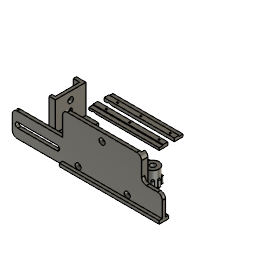
camera_steady (Autodesk Fusion 360 design; units mm, degrees)
Autodesk Fusion 360 part; units mm, degrees
note: some values were not read from the file. Chosen so that the rebuilt part matches the saved one: which face or edge a step refers to; which sketch regions a step uses; which pieces of a blend or face edit are solid.
sketch "Sketch1" plane through (0, 0, 0) normal (0, 0, 1) x (1, 0, 0)
  line L0 (-42, 80) -> (-26, 80)
  line L1 (0, 50) -> (118, 50)
  line L2 (118, 50) -> (118, 62)
  line L3 (118, 62) -> (-70, 62)
  line L4 (-70, 62) -> (-70, 54)
  line L5 (-7, 54) -> (-7, 62)
  line L6 (-3, 54) -> (-3, 62)
  line L7 (88, 50) -> (88, 62)
  line L8 (92, 50) -> (92, 62)
  line L9 (118, 58) -> (-70.000001, 58)
  line L10 (-70, 54) -> (98, 54)
  line L11 (-42, 118.4) -> (-42, 80)
  line L12 (-26, 118.4) -> (-26, 80)
  line L13 (-42, 118.4) -> (-26, 118.4)
  line L14 (-42, 118.4) -> (-46, 118.4)
  line L15 (-42, 80) -> (-46, 80)
  line L16 (-46, 114.4) -> (-46, 84)
  line L17 (-46, 118.4) -> (-54, 118.4)
  line L18 (-46, 80) -> (-50, 80)
  line L19 (-46, 114.4) -> (-54, 114.4)
  line L20 (-46, 80) -> (-50, 80)
  line L21 (-46, 84) -> (-50, 84)
  line L22 (-54, 118.4) -> (-54, 114.4)
  line L23 (-50, 80) -> (-50, 84)
  line L24 (25, 80) -> (50, 80)
  line L25 (50, 80) -> (50, 110)
  line L26 (50, 110) -> (25, 110)
  line L27 (25, 84) -> (50, 84)
  circle A0 centre (35, 95) radius 3.2
  circle A1 centre (35, 95) radius 10.7
  line L28 (-50, 130) -> (36, 130)
  line L29 (36, 141) -> (-50, 141)
  line L30 (-50, 141) -> (-50, 130)
  line L31 (-50, 135) -> (36, 135)
  circle A2 centre (-36.000001, 138.000002) radius 1.1
  circle A3 centre (-7, 138) radius 1.1
  circle A4 centre (30, 138.000002) radius 1.1
  line L32 (-50.000001, 145.000002) -> (35.000001, 145.000002) construction
  circle A5 centre (30, 152.000002) radius 1.1
  line L33 (-50, 149.000004) -> (-50, 160.000004)
  line L34 (-50, 155.000004) -> (36, 155.000004)
  line L35 (36, 149.000004) -> (-50, 149.000004)
  circle A6 centre (-36.000001, 152.000002) radius 1.1
  line L36 (-50, 160.000004) -> (36, 160.000004)
  circle A7 centre (-7, 152.000004) radius 1.1
  line L37 (-44, 141) -> (-44, 130)
  line L38 (-44, 149.000004) -> (-44, 160.000004)
  line L39 (98, 54) -> (118, 54)
  line L40 (20.07966, 95) -> (20.07966, 110)
  line L41 (20.07966, 95) -> (20.07966, 80)
  line L42 (25, 80) -> (20.07966, 80)
  line L43 (25, 84) -> (20.07966, 84)
  line L44 (25, 110) -> (20.07966, 110)
  line L45 (-7, 54) -> (-7, 50)
  line L46 (-7, 50) -> (0, 50)
  circle A8 centre (70.000001, 90.000001) radius 3.3
  circle A9 centre (70.000001, 90.000001) radius 8
  arc A10 (65.498572, 96.613407) -> (63.386595, 94.50143) centre (64.343147, 95.656856) ccw
  arc A11 (71.493395, 97.859376) -> (68.506607, 97.859376) centre (70.000001, 98.000001) ccw
  arc A12 (76.613407, 94.50143) -> (74.50143, 96.613407) centre (75.656855, 95.656856) ccw
  arc A13 (77.859376, 88.506608) -> (77.859376, 91.493395) centre (78.000001, 90.000001) ccw
  arc A14 (74.50143, 83.386595) -> (76.613407, 85.498573) centre (75.656855, 84.343147) ccw
  arc A15 (68.506607, 82.140626) -> (71.493395, 82.140626) centre (70.000001, 82.000001) ccw
  arc A16 (63.386595, 85.498573) -> (65.498572, 83.386595) centre (64.343147, 84.343147) ccw
  arc A17 (62.140626, 91.493395) -> (62.140626, 88.506608) centre (62.000001, 90.000001) ccw
  line L47 (38, 160.000004) -> (38, 149.000004)
  line L48 (36, 149.000004) -> (38, 149.000004)
  line L49 (36, 160.000004) -> (38, 160.000004)
  line L50 (36, 155.000004) -> (38.000001, 155.000004)
  line L51 (38, 130) -> (38, 141)
  line L52 (36, 130) -> (38, 130)
  line L53 (36, 141) -> (38, 141)
  line L54 (36, 135) -> (38, 135)
  line L55 (34.999999, 89.157067) -> (29.939871, 92.078534)
  line L56 (29.939871, 92.078534) -> (29.939872, 97.921467)
  line L57 (29.939872, 97.921467) -> (35.000001, 100.842933)
  line L58 (35.000001, 100.842933) -> (40.060129, 97.921466)
  line L59 (40.060129, 97.921466) -> (40.060128, 92.078533)
  line L60 (40.060128, 92.078533) -> (34.999999, 89.157067)
  point P0 (35, 95)
  point P1 (-7, 141)
  point P2 (-7, 138)
  point P3 (-36.000001, 138.000002)
  point P4 (30, 138.000002)
  point P5 (30, 152.000002)
  point P6 (-7, 152.000004)
  point P7 (-36.000001, 152.000002)
  point P8 (-7, 149.000004)
  point P9 (-44, 130)
  point P10 (-44, 149.000004)
  point P11 (70.000001, 90.000001)
  point P12 (70.000001, 98.000001)
  dimension "d43" = 168
  dimension "d54" = 38.4
  dimension "d64" = 4
  dimension "d69" = 4
  dimension "d81" = 6.4
  dimension "d82" = 21.4
  dimension "d92" = 86
  dimension "d93" = 11
  dimension "d100" = 2.2
  dimension "d101" = 2.2
  dimension "d102" = 2.2
  dimension "d103" = 11
  dimension "d118" = 6.6
  dimension "d119" = 16
  dimension "d120" = 3
  dimension "d122" = 360
  constraint horizontal L0
  constraint horizontal L1
  constraint vertical L2
  constraint horizontal L3
  constraint vertical L4
  constraint coincident L3 L5.end
  constraint perpendicular L3 L5
  constraint coincident L3 L6.end
  constraint perpendicular L3 L6
  constraint coincident L3 L7.end
  constraint perpendicular L3 L7
  constraint coincident L3 L8.end
  constraint perpendicular L3 L8
  constraint coincident L1 L7.start
  constraint coincident L1 L8.start
  constraint horizontal L9
  constraint horizontal L10
  constraint vertical L11
  constraint vertical L12
  constraint coincident L10 L5.start
  constraint perpendicular L12 L13
  constraint perpendicular L11 L14
  constraint perpendicular L11 L15
  constraint perpendicular L16 L17
  constraint perpendicular L16 L18
  constraint perpendicular L19 L22
  constraint perpendicular L21 L23
  constraint horizontal L24
  constraint vertical L25
  constraint horizontal L26
  constraint horizontal L27
  constraint coincident P0 A0.centre
  constraint concentric A0 A1
  constraint horizontal L28
  constraint horizontal L29
  constraint vertical L30
  constraint horizontal L31
  constraint midpoint L29 P1
  constraint coincident P2 A3.centre
  constraint horizontal L32
  constraint symmetric A2 L32 A6
  constraint symmetric A3 L32 A7
  constraint symmetric A4 L32 A5
  constraint vertical L37
  constraint coincident P9 L37.end
  constraint coincident L2 L39.end
  constraint perpendicular L2 L39
  constraint perpendicular L41 L42
  constraint perpendicular L41 L43
  constraint perpendicular L40 L44
  constraint perpendicular L10 L45
  constraint perpendicular L6 L46
  constraint coincident L10 L6.start
  constraint concentric A8 A9
  constraint perpendicular L47 L48
  constraint perpendicular L47 L49
  constraint perpendicular L47 L50
  constraint vertical L51
  constraint perpendicular L51 L52
  constraint perpendicular L51 L53
  constraint coincident L51 L54.end
  constraint perpendicular L51 L54
  measures "d43" distance of L10.end L4.end
  measures "d54" distance of L0.start L11.start
  measures "d64" distance of L0.start L15.end
  measures "d69" distance of L21.end L16.end
  measures "d81" diameter of A0
  measures "d82" diameter of A1
  measures "d92" distance of L28.start L28.end
  measures "d93" distance of L28.start L29.end
  measures "d100" diameter of A2
  measures "d101" diameter of A3
  measures "d102" diameter of A4
  measures "d103" distance of P9 L37.start
  measures "d118" diameter of A8
  measures "d119" diameter of A9
  measures "d120" diameter of A11
extrude "Extrude15" add sketch "Sketch1" along normal blind 4 contours L1 L7 L10 L45 L46 | L1 L7 L8 L10 | L1 L2 L8 L10 L39 | L6 L7 L9 L10 picked at (28.333333, 52.666667) picked at (90.666667, 51.333333) picked at (102.666667, 51.333333) picked at (57.666667, 55.333333) makes body 1
extrude "Extrude16" add sketch "Sketch1" along normal blind 30 contours L4 L5 L9 L10 | L2 L8 L9 L10 L39 picked at (-49, 56.666667) picked at (102.666667, 56.666667) bodies 1
extrude "Extrude31" add sketch "Sketch1" along normal blind 60 contours L6 L7 L9 L10 | L7 L8 L9 L10 | L5 L6 L9 L10 | L3 L7 L8 L9 | L3 L5 L6 L9 picked at (57.666667, 55.333333) picked at (89.333333, 56.666667) picked at (-5.666667, 55.333333) picked at (89.333333, 60.666667) picked at (-5.666667, 59.333333) bodies 1
extrude "Extrude17" add sketch "Sketch1" along normal blind 4 contours L3 L6 L7 L9 | L3 L4 L5 L9 | L2 L3 L8 L9 picked at (57.666667, 59.333333) picked at (-49, 59.333333) picked at (100.666667, 59.333333) bodies 1
sketch "Sketch2" plane through (0, 54, 0) normal (0, -1, 0) x (1, 0, 0)
  line L0 (118, 30) -> (92, 30)
  line L1 (-70, 30) -> (-70, 0)
  line L2 (-70, 0) -> (-7, 0)
  line L3 (-7, 4) -> (118, 4)
  line L4 (92, 30) -> (92, 60)
  line L5 (92, 60) -> (-7, 60)
  line L6 (-7, 60) -> (-7, 30)
  arc A0 (-63, 18.2) -> (-62.999999, 11.8) centre (-63, 15) ccw
  line L7 (-11, 15) -> (-63, 15) construction
  line L8 (118, 4) -> (118, 30)
  line L9 (-7, 0) -> (-7, 4)
  line L10 (-7, 30) -> (-70, 30)
  line L11 (-63, 18.2) -> (-13.998804, 18.2)
  line L12 (-62.999999, 11.8) -> (-14, 11.8)
  line L13 (-7, 4) -> (-7, 60)
  line L14 (-4, 4) -> (-4, 60)
  line L15 (-4, 4) -> (-4, 60)
  arc A1 (-14, 11.8) -> (-14.001196, 18.2) centre (-14, 15) ccw
  circle A2 centre (74, 8) radius 1.3
  circle A3 centre (42.5, 50) radius 1.3
  circle A4 centre (12.5, 8) radius 1.3
  point P0 (-70, 15)
  point P1 (-225, 15)
  point P2 (-285, 15)
  point P3 (-37, 15)
  point P4 (-37, 15)
  point P5 (-21, 15)
  point P6 (-63, 15)
  point P7 (-14, 15)
  point P8 (42.5, 50)
  point P9 (42.5, 50)
  point P10 (49.314107, -3.66554)
  point P11 (12.5, 8)
  point P12 (74, 8)
  dimension "d115" = 6.4
  dimension "d135" = 6.4
  dimension "d147" = 2.6
  dimension "d148" = 2.6
  dimension "d149" = 2.6
  constraint midpoint L1 P0
  constraint horizontal L7
  constraint coincident P4 P3
  constraint midpoint L7 P4
  constraint coincident P6 A0.centre
  constraint parallel L10 L11
  constraint parallel L7 L12
  constraint coincident L7 P7
  constraint coincident P7 A1.centre
  constraint coincident P12 A2.centre
  constraint coincident P9 P8
  constraint coincident P11 A4.centre
  measures "d115" diameter of A0
  measures "d135" diameter of A1
  measures "d147" diameter of A2
  measures "d148" diameter of A3
  measures "d149" diameter of A4
extrude "Extrude18" cut sketch "Sketch2" against normal blind 4 contours A0 L11 L12 A1 | A2 | A3 | A4 picked at (-30.333732, 13.933333) picked at (73.641963, 7.626725) picked at (41.878655, 49.935415) picked at (12.914082, 7.872273) bodies 1
chamfer "Chamfer1" distance 2.4 angle 45 3 edges at (41.287974, 54, 50.4701) (11.287974, 54, 8.4701) (72.787974, 54, 8.4701) on bodies 1
fillet "Fillet1" radius 6 6 edges at (92, 58, 60) (-7, 58, 60) (118, 56, 30) (92, 56, 30) (-70.000001, 56, 30) (-70, 58, 0) on bodies 1
extrude "Extrude22" add sketch "Sketch1" along normal blind 4 separate body contours L0 L11 L12 L13 picked at (-36.666667, 105.6) makes body 2
extrude "Extrude23" add sketch "Sketch1" along normal blind 40 contours L11 L14 L15 L16 L17 L18 L19 L20 L21 L22 L23 picked at (-43.333333, 94.133333) bodies 2
sketch "Sketch4" plane through (-42, 0, 0) normal (1, 0, 0) x (0, 1, 0)
  line L0 (80, 4) -> (118.4, 4)
  line L1 (118.4, 4) -> (118.4, 40)
  line L2 (118.4, 40) -> (80, 40)
  line L3 (80, 40) -> (80, 4)
  circle A0 centre (99.2, 30) radius 3.4
  circle A1 centre (99.2, 14) radius 3.4
  point P0 (99.2, 30)
  point P1 (99.2, 14)
  dimension "d87" = 6.8
  dimension "d88" = 6.8
  constraint coincident P0 A0.centre
  constraint coincident P1 A1.centre
  measures "d87" diameter of A0
  measures "d88" diameter of A1
extrude "Extrude24" cut sketch "Sketch4" against normal blind 4 contours A0 | A1 picked at (97.994631, 30.96125) picked at (97.597353, 13.411499) bodies 2
extrude "Extrude25" add sketch "Sketch1" along normal blind 4 separate body contours L25 L26 L27 L40 L41 L43 L44 picked at (21.839651, 101.547519) makes body 3
extrude "Extrude26" add sketch "Sketch1" along normal blind 9 contours A1 | L55 L56 L57 L58 L59 L60 picked at (31.529958, 101.010291) picked at (30.559914, 95) bodies 3
extrude "Extrude27" add sketch "Sketch1" along normal blind 9 contours L55 L56 L57 L58 L59 L60 picked at (30.559914, 95) bodies 3
sketch "Sketch7" plane through (0, 0, 9) normal (0, 0, 1) x (-1, 0, 0)
  circle A0 centre (-35, -95) radius 10.7
  circle A1 centre (-35, -95) radius 3.2
  line L0 (-40.060128, -92.078533) -> (-34.999999, -89.157067)
  line L1 (-34.999999, -89.157067) -> (-29.939871, -92.078534)
  line L2 (-29.939871, -92.078534) -> (-29.939872, -97.921467)
  line L3 (-29.939872, -97.921467) -> (-35.000001, -100.842933)
  line L4 (-35.000001, -100.842933) -> (-40.060129, -97.921466)
  line L5 (-40.060129, -97.921466) -> (-40.060128, -92.078533)
extrude "Extrude36" cut sketch "Sketch7" against normal blind 5 contours L0 L1 L2 L3 L4 L5 picked at (-37.220043, -98.845227) bodies 3
extrude "Extrude28" add sketch "Sketch1" along normal blind 4 separate body contours L29 L30 L31 L37 | L29 L31 L37 L51 L53 L54 | L33 L34 L35 L38 | L34 L35 L38 L47 L48 L50 picked at (-48, 139) picked at (-41.7, 138.000001) picked at (-48, 153.000004) picked at (-41.7, 152.000004) makes body 4 at (-45.7, 138.000001, 0) makes body 5 at (-45.7, 152.000004, 0)
extrude "Extrude29" add sketch "Sketch1" along normal blind 3 contours L28 L30 L31 L37 | L28 L31 L37 L51 L52 L54 | L29 L30 L31 L37 | L33 L34 L36 L38 | L34 L36 L38 L47 L49 L50 picked at (-48, 133.333333) picked at (-17.333333, 133.333333) picked at (-48, 139) picked at (-48, 158.333338) picked at (-17.333333, 158.333338) bodies 4 5
sketch "Sketch5" plane through (0, 130, 0) normal (0, -1, 0) x (1, 0, 0)
  line L0 (-50, 0) -> (38, 0)
  line L1 (38, 3) -> (-50, 3)
  line L2 (-50, 3) -> (-50, 0)
  arc A0 (-41.757859, 0) -> (-46.229995, 0) centre (-43.993927, -2) ccw
  line L3 (38, 0) -> (38, 3)
  point P0 (-41.757859, 0)
  dimension "d107" = 6
  measures "d107" diameter of A0
extrude "Extrude30" cut sketch "Sketch5" against normal blind 30 contours L0 A0 picked at (-44.402176, 0.246204) bodies 4 5
fillet "Fillet2" radius 2 4 edges at (50, 110, 2) (50, 84, 2) (20.07966, 110, 2) (20.07966, 84, 2) on bodies 3
extrude "Extrude32" add sketch "Sketch1" along normal blind 20 separate body contours A9 picked at (73.236744, 84.454625) makes body 6
extrude "Extrude33" add sketch "Sketch1" along normal blind 10 contours A9 A13 | A9 A12 | A9 A14 | A9 A11 | A9 A15 | A9 A10 | A9 A16 | A9 A17 picked at (78.462394, 89.656178) picked at (76.027665, 95.976531) picked at (76.027665, 84.023471) picked at (70.036158, 98.488248) picked at (69.963844, 81.511754) picked at (63.972337, 95.976531) picked at (63.972337, 84.023471) picked at (61.511754, 89.963844) bodies 6
fillet "Fillet3" radius 1 8 edges at (76.717516, 96.717516, 10) (70.000001, 99.500001, 10) (63.282487, 96.717516, 10) (60.500001, 90.000001, 10) (63.282487, 83.282487, 10) (70.000001, 80.500001, 10) (76.717516, 83.282487, 10) (79.500001, 90.000001, 10) on bodies 6
fillet "Fillet4" radius 1 16 edges at (79.500001, 90.000001, 0) (76.717516, 96.717516, 0) (70.000001, 99.500001, 0) (63.282487, 96.717516, 0) (60.500001, 90.000001, 0) (63.282487, 83.282487, 0) (70.000001, 80.500001, 0) (76.717516, 83.282487, 0) (77.391037, 93.061469, 0) (73.061469, 97.391038, 0) (66.938534, 97.391038, 0) (62.608965, 93.061469, 0) (62.608965, 86.938534, 0) (66.938534, 82.608965, 0) (73.061469, 82.608965, 0) (77.391037, 86.938534, 0) on bodies 6
sketch "Sketch6" plane through (0, 0, 0) normal (0, 0, 1) x (1, 0, 0)
  line L0 (75.070128, 92.927241) -> (70.000001, 95.85448)
  line L1 (70.000001, 95.85448) -> (64.929874, 92.927241)
  line L2 (64.929874, 92.927241) -> (64.929874, 87.072762)
  line L3 (64.929874, 87.072762) -> (70.000001, 84.145523)
  line L4 (70.000001, 84.145523) -> (75.070128, 87.072762)
  line L5 (75.070128, 92.927241) -> (75.070128, 87.072762)
  point P0 (70.000001, 90.000001)
extrude "Extrude34" cut sketch "Sketch6" along normal blind 4 bodies 6
